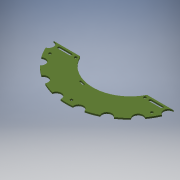
# Autodesk Inventor part: Board_Shape
Saved by Autodesk Inventor 2016 (Build 200138000, 138)
## iProperties
Created: 2015-08-05
Part Number: Board_Shape
Material: Generic
Document SubType Name: Modeling
Designer: 3DPrinterUser
Density: 1 g/cm^3
Appearance: Olive Green
Author: 3DPrinterUser
Autodesk Inventor part; units mm, degrees
ref_plane "YZ Plane" through (0, 0, 0) normal (1, 0, 0) x (0, 1, 0)
ref_plane "XZ Plane" through (0, 0, 0) normal (0, 1, 0) x (-1, 0, 0)
ref_plane "XY Plane" through (0, 0, 0) normal (0, 0, 1) x (1, 0, 0)
sketch "Sketch1" plane through (0, 0, 0) normal (0, 0, 1) x (1, 0, 0)
  circle A0 centre (46.9462, 34.742) radius 1.05 projected
  circle A1 centre (53.415, 34.1058) radius 1.05 projected
  circle A2 centre (-46.9442, -34.742) radius 1.05 construction
  circle A3 centre (-53.413, -34.1058) radius 1.05 construction
  arc A4 (72.8682, -20.1426) -> (68.7671, -31.41) centre (71.0414, -25.8577) ccw projected
  arc A5 (72.8682, -20.1426) -> (72.8688, 20.1405) centre (0.001, 0) ccw projected
  arc A6 (68.768, 31.408) -> (72.8688, 20.1405) centre (71.0421, 25.8557) ccw projected
  arc A7 (68.768, 31.408) -> (61.5859, 43.8482) centre (0.001, 0) ccw projected
  arc A8 (53.8786, 53.0336) -> (61.5859, 43.8482) centre (57.9147, 48.5939) ccw projected
  arc A9 (53.8786, 53.0336) -> (42.8749, 62.2671) centre (0.001, 0) ccw projected
  arc A10 (32.4909, 68.2625) -> (42.8749, 62.2671) centre (37.8019, 65.471) ccw projected
  arc A11 (32.4909, 68.2625) -> (18.9927, 73.1756) centre (0.001, 0) ccw projected
  arc A12 (7.1843, 75.258) -> (18.9927, 73.1756) centre (13.1299, 74.4513) ccw projected
  arc A13 (7.1843, 75.258) -> (-7.1802, 75.2582) centre (0.001, 0) ccw projected
  arc A14 (-18.9886, 73.1762) -> (-7.1802, 75.2582) centre (-13.1257, 74.4517) ccw projected
  arc A15 (-18.9886, 73.1762) -> (-32.4869, 68.2634) centre (0.001, 0) ccw projected
  arc A16 (-42.8711, 62.2683) -> (-32.4869, 68.2634) centre (-37.7981, 65.4721) ccw projected
  arc A17 (-42.8711, 62.2683) -> (-53.8751, 53.0351) centre (0.001, 0) ccw projected
  arc A18 (-61.5826, 43.8499) -> (-53.8751, 53.0351) centre (-57.9113, 48.5956) ccw projected
  arc A19 (-61.5826, 43.8499) -> (-68.7651, 31.41) centre (0.001, 0) ccw projected
  arc A20 (-72.8662, 20.1426) -> (-68.7651, 31.41) centre (-71.0394, 25.8577) ccw projected
  arc A21 (-72.8662, 20.1426) -> (-72.8668, -20.1405) centre (0.001, 0) ccw projected
  arc A22 (-68.766, -31.408) -> (-72.8668, -20.1405) centre (-71.0401, -25.8557) ccw projected
  arc A23 (-68.766, -31.408) -> (-61.5839, -43.8482) centre (0.001, 0) ccw projected
  arc A24 (-53.8766, -53.0336) -> (-61.5839, -43.8482) centre (-57.9127, -48.5939) ccw projected
  arc A25 (-53.8766, -53.0336) -> (-42.8729, -62.2671) centre (0.001, 0) ccw projected
  arc A26 (-32.4889, -68.2625) -> (-42.8729, -62.2671) centre (-37.7999, -65.471) ccw projected
  arc A27 (-32.4889, -68.2625) -> (-18.9907, -73.1756) centre (0.001, 0) ccw projected
  arc A28 (-7.1823, -75.258) -> (-18.9907, -73.1756) centre (-13.1279, -74.4513) ccw projected
  arc A29 (-7.1823, -75.258) -> (7.1822, -75.2582) centre (0.001, 0) ccw projected
  arc A30 (18.9906, -73.1762) -> (7.1822, -75.2582) centre (13.1277, -74.4517) ccw projected
  arc A31 (18.9906, -73.1762) -> (32.4889, -68.2634) centre (0.001, 0) ccw projected
  arc A32 (42.8731, -62.2683) -> (32.4889, -68.2634) centre (37.8001, -65.4721) ccw projected
  arc A33 (42.8731, -62.2683) -> (53.8771, -53.0351) centre (0.001, 0) ccw projected
  arc A34 (61.5846, -43.8499) -> (53.8771, -53.0351) centre (57.9133, -48.5956) ccw projected
  arc A35 (61.5846, -43.8499) -> (68.7671, -31.41) centre (0.001, 0) ccw projected
  circle A36 centre (0.001, 0) radius 44.3 projected
  circle A37 centre (-69.9492, -11.499) radius 1.3 projected
  circle A38 centre (-46.9488, 11.5007) radius 1.3 projected
  circle A39 centre (69.9508, -11.501) radius 1.3 projected
  circle A40 centre (46.9512, 11.4993) radius 1.3 projected
  circle A41 centre (69.9512, 11.499) radius 1.3 projected
  circle A42 centre (46.9508, -11.5007) radius 1.3 projected
  circle A43 centre (-69.9488, 11.501) radius 1.3 projected
  circle A44 centre (-46.9492, -11.4993) radius 1.3 projected
  circle A45 centre (-58.449, 0.0008) radius 11.5 projected
  circle A46 centre (58.451, -0.0008) radius 11.5 projected
  circle A47 centre (60.2759, -34.8009) radius 1.55 projected
  circle A48 centre (44.7383, -53.3173) radius 1.55 projected
  circle A49 centre (16.1779, -44.4477) radius 1.55 projected
  circle A50 centre (0, -69.6) radius 1.55 projected
  circle A51 centre (-23.8045, -65.4023) radius 1.55 projected
  circle A52 centre (-30.4034, -36.2335) radius 1.55 projected
  circle A53 centre (-60.2749, -34.7991) radius 1.55 projected
  circle A54 centre (60.2769, 34.7991) radius 1.55 projected
  circle A55 centre (44.7398, 53.3161) radius 1.55 projected
  circle A56 centre (23.8065, 65.4023) radius 1.55 projected
  circle A57 centre (-40.9617, 23.6506) radius 1.55 projected
  circle A58 centre (-30.4023, 36.2343) radius 1.55 projected
  circle A59 centre (-16.1759, 44.4477) radius 1.55 projected
  circle A60 centre (0.0017, 47.3) radius 1.55 projected
  circle A61 centre (0.002, 69.6) radius 1.55 projected
  circle A62 centre (-23.8027, 65.4029) radius 1.55 projected
  circle A63 centre (-44.7363, 53.3173) radius 1.55 projected
  circle A64 centre (-60.2739, 34.8009) radius 1.55 projected
  circle A65 centre (16.1792, 44.4472) radius 1.55 projected
  circle A66 centre (30.4054, 36.2335) radius 1.55 projected
  circle A67 centre (40.9643, 23.6494) radius 1.55 projected
  circle A68 centre (-40.9623, -23.6494) radius 1.55 projected
  circle A69 centre (-44.7378, -53.3161) radius 1.55 projected
  circle A70 centre (-16.1772, -44.4472) radius 1.55 projected
  circle A71 centre (0.0003, -47.3) radius 1.55 projected
  circle A72 centre (23.8047, -65.4029) radius 1.55 projected
  circle A73 centre (30.4043, -36.2343) radius 1.55 projected
  circle A74 centre (40.9637, -23.6506) radius 1.55 projected
  line L0 (58.451, 0) -> (0.001, 0) construction
  line L1 (71.0414, -19.8577) -> (39.601, -19.8577)
  line L2 (-71.0401, -19.8557) -> (-39.6, -19.8557)
  point P0 (0, 0)
  constraints: 6 end point, 4 point on circle, 2 parallel, 2 tangent, 1 horizontal
extrude "Extrusion1" add sketch "Sketch1" along normal blind 1.75 contours A4 A35 A34 A33 A32 A31 A30 A29 A28 A27 A26 A25 A24 A23 A22 L2 A36 L1
sketch "Sketch2" plane through (0, 0, 1.75) normal (0, 0, 1) x (1, 0, 0)
  circle A0 centre (-30.4034, -36.2335) radius 1.55 projected
  circle A1 centre (-44.7378, -53.3161) radius 1.55 projected
  circle A2 centre (-23.8045, -65.4023) radius 1.55 projected
  circle A3 centre (-16.1772, -44.4472) radius 1.55 projected
  circle A4 centre (16.1779, -44.4477) radius 1.55 projected
  circle A5 centre (23.8047, -65.4029) radius 1.55 projected
  circle A6 centre (44.7383, -53.3173) radius 1.55 projected
  circle A7 centre (30.4043, -36.2343) radius 1.55 projected
  circle A8 centre (0.0003, -47.3) radius 1.55 projected
  point P0 (0, 0)
extrude "Extrusion2" add sketch "Sketch2" against normal up to surface (1.75 mm away)
sketch "Sketch3" plane through (0, 0, 1.75) normal (0, 0, 1) x (1, 0, 0)
  line L0 (-60.9088, -23.5183) -> (-47.1121, -23.5183) construction
  line L1 (-60.9088, -25.0183) -> (-47.1121, -25.0183)
  line L2 (-47.1121, -22.0183) -> (-60.9088, -22.0183)
  arc A0 (-60.9088, -22.0183) -> (-60.9088, -25.0183) centre (-60.9088, -23.5183) ccw
  arc A1 (-47.1121, -25.0183) -> (-47.1121, -22.0183) centre (-47.1121, -23.5183) ccw
  line L3 (-60.9088, -23.5183) -> (-65.5141, -23.5183) construction
  arc A2 (-68.766, -31.408) -> (-71.0401, -19.8557) centre (-71.0401, -25.8557) ccw projected
  line L4 (-47.1121, -23.5183) -> (-42.5068, -23.5183) construction
  circle A3 centre (-40.9623, -23.6494) radius 1.55 projected
  point P0 (0, 0)
  point P1 (-54.0105, -23.5183)
  dimension "d4" = 3
  constraints: 12 end point, 5 point on circle, 4 tangent, 2 centre point, 2 horizontal, 1 collinear, 1 midpoint, 1 parallel, 1 point on line, 2 other
  measures "d4" diameter of A1
extrude "Extrusion3" cut sketch "Sketch3" against normal up to surface (1.75 mm away) contours A0 L2 A1 L1
mirror "Mirror1" about plane through (0, 0, 0) normal (1, 0, 0) of "Extrusion3"
sketch "Sketch4" plane through (0, 0, 1.75) normal (0, 0, 1) x (1, 0, 0)
  line L0 (13.6094, 45.369) -> (8.7511, 46.5508) construction
  line L1 (13.8458, 46.3407) -> (8.9875, 47.5225)
  line L2 (8.5148, 45.5792) -> (13.3731, 44.3973)
  arc A0 (13.3731, 44.3973) -> (13.8458, 46.3407) centre (13.6094, 45.369) ccw
  arc A1 (8.9875, 47.5225) -> (8.5148, 45.5792) centre (8.7511, 46.5508) ccw
  circle A2 centre (0, 0) radius 47.3002 construction
  arc A3 (-39.6, -19.8557) -> (39.601, -19.8577) centre (0.001, 0) ccw projected
  point P0 (11.1803, 45.9599)
  dimension "d7" = 2
  dimension "d8" = 5
  dimension "d9" = 2
  constraints: 8 end point, 4 point on circle, 4 tangent, 2 centre point, 1 coincident, 1 midpoint, 1 parallel, 4 other
  measures "d7" diameter of A1
  measures "d8" distance of L0.start L0.end
  measures "d9" distance edge to line of A3 L2
extrude "Extrusion4" cut sketch "Sketch4" against normal up to surface (1.75 mm away)
equation "\"d0\" = board_height"
equation "\"d2\" = board_height"
equation "\"d5\" = board_height"
equation "\"d10\" = board_height"
equation "\"board_height\" = 1.75"
body "Solid1"
